Autodesk Fusion 360 part; units mm, degrees
(part 7 of 7)
  spline S53 degree 5 poles (-12.3121, 39.5225) (-12.3132, 39.5068) (-12.3154, 39.4756) (-12.3186, 39.4286) (-12.3227, 39.3661) (-12.3275, 39.288) (-12.332, 39.21) (-12.3361, 39.132) (-12.34, 39.054) (-12.3435, 38.9761) (-12.3467, 38.8983) (-12.3495, 38.8205) (-12.3521, 38.7428) (-12.3543, 38.6651) (-12.3562, 38.5875) (-12.3578, 38.51) (-12.359, 38.4325) (-12.3599, 38.3551) (-12.3605, 38.2777) (-12.3607, 38.2004) (-12.3606, 38.1232) (-12.3601, 38.0461) (-12.3593, 37.969) (-12.3581, 37.892) (-12.3566, 37.8151) (-12.3548, 37.7383) (-12.3525, 37.6615) (-12.35, 37.5848) (-12.347, 37.5082) (-12.3437, 37.4317) (-12.34, 37.3553) (-12.336, 37.2789) (-12.3315, 37.2027) (-12.3267, 37.1265) (-12.3215, 37.0505) (-12.3159, 36.9745) (-12.3099, 36.8987) (-12.3036, 36.8229) (-12.2968, 36.7473) (-12.2896, 36.6717) (-12.282, 36.5963) (-12.274, 36.521) (-12.2656, 36.4458) (-12.2567, 36.3708) (-12.2474, 36.2958) (-12.2377, 36.221) (-12.2275, 36.1463) (-12.2169, 36.0718) (-12.2059, 35.9974) (-12.1944, 35.9231) (-12.1823, 35.849) (-12.1698, 35.775) (-12.1568, 35.7013) (-12.1432, 35.6277) (-12.1291, 35.5542) (-12.1145, 35.481) (-12.0994, 35.4079) (-12.0838, 35.3349) (-12.0678, 35.2622) (-12.0511, 35.1896) (-12.0338, 35.1173) (-12.0157, 35.0453) (-11.9967, 34.9736) (-11.9769, 34.9022) (-11.9563, 34.8311) (-11.9352, 34.7603) (-11.9136, 34.6896) (-11.8917, 34.619) (-11.8692, 34.5488) (-11.8455, 34.4789) (-11.8201, 34.4098) (-11.7979, 34.3554) (-11.7798, 34.3151) (-11.7671, 34.2886) (-11.7607, 34.2754) knots -1 -1 -1 -1 -1 -1 -0.98571429 -0.97142857 -0.95714286 -0.94285714 -0.92857143 -0.91428571 -0.9 -0.88571429 -0.87142857 -0.85714286 -0.84285714 -0.82857143 -0.81428571 -0.8 -0.78571429 -0.77142857 -0.75714286 -0.74285714 -0.72857143 -0.71428571 -0.7 -0.68571429 -0.67142857 -0.65714286 -0.64285714 -0.62857143 -0.61428571 -0.6 -0.58571429 -0.57142857 -0.55714286 -0.54285714 -0.52857143 -0.51428571 -0.5 -0.48571429 -0.47142857 -0.45714286 -0.44285714 -0.42857143 -0.41428571 -0.4 -0.38571429 -0.37142857 -0.35714286 -0.34285714 -0.32857143 -0.31428571 -0.3 -0.28571429 -0.27142857 -0.25714286 -0.24285714 -0.22857143 -0.21428571 -0.2 -0.18571429 -0.17142857 -0.15714286 -0.14285714 -0.12857143 -0.11428571 -0.1 -0.08571429 -0.07142857 -0.05714286 -0.04285714 -0.02857143 -0.01428571 0 0 0 0 0 0
  line L53 (-11.7607, 34.2754) -> (-11.6323, 34.014)
  arc A108 (-11.7749, 33.5903) -> (-11.6323, 34.014) centre (-11.9173, 33.8741) ccw
  arc A109 (-11.7749, 33.5903) -> (-13.4852, 32.6761) centre (5.08, 0) ccw
  arc A110 (-13.9168, 32.7929) -> (-13.4852, 32.6761) centre (-13.6421, 32.9522) ccw
  line L54 (-13.9168, 32.7929) -> (-14.0628, 33.0449)
  spline S54 degree 5 poles (-14.0628, 33.0449) (-14.0701, 33.0576) (-14.0852, 33.0829) (-14.1086, 33.1203) (-14.1415, 33.169) (-14.1849, 33.2285) (-14.2298, 33.287) (-14.2757, 33.3448) (-14.3222, 33.4022) (-14.369, 33.4594) (-14.4162, 33.5163) (-14.4638, 33.5729) (-14.5121, 33.6291) (-14.5612, 33.6847) (-14.611, 33.7397) (-14.6615, 33.7943) (-14.7126, 33.8485) (-14.7642, 33.9022) (-14.8162, 33.9557) (-14.8686, 34.0089) (-14.9214, 34.0617) (-14.9746, 34.1142) (-15.0283, 34.1664) (-15.0824, 34.2183) (-15.1369, 34.2698) (-15.1919, 34.3209) (-15.2472, 34.3717) (-15.303, 34.4223) (-15.359, 34.4725) (-15.4155, 34.5225) (-15.4723, 34.5721) (-15.5294, 34.6215) (-15.5869, 34.6706) (-15.6447, 34.7193) (-15.7029, 34.7678) (-15.7614, 34.816) (-15.8202, 34.864) (-15.8794, 34.9116) (-15.9388, 34.959) (-15.9985, 35.0061) (-16.0586, 35.053) (-16.1189, 35.0995) (-16.1796, 35.1459) (-16.2405, 35.1919) (-16.3017, 35.2377) (-16.3632, 35.2832) (-16.425, 35.3285) (-16.4871, 35.3735) (-16.5494, 35.4182) (-16.612, 35.4627) (-16.6748, 35.507) (-16.738, 35.551) (-16.8013, 35.5947) (-16.865, 35.6382) (-16.9288, 35.6814) (-16.993, 35.7244) (-17.0574, 35.7672) (-17.122, 35.8097) (-17.1869, 35.852) (-17.252, 35.894) (-17.3173, 35.9358) (-17.3829, 35.9773) (-17.4487, 36.0186) (-17.5148, 36.0597) (-17.581, 36.1005) (-17.6475, 36.1411) (-17.7142, 36.1814) (-17.7812, 36.2215) (-17.8483, 36.2614) (-17.9157, 36.3011) (-17.9833, 36.3405) (-18.0376, 36.3718) (-18.0783, 36.3952) (-18.1056, 36.4108) (-18.1192, 36.4185) knots 0 0 0 0 0 0 0.01428571 0.02857143 0.04285714 0.05714286 0.07142857 0.08571429 0.1 0.11428571 0.12857143 0.14285714 0.15714286 0.17142857 0.18571429 0.2 0.21428571 0.22857143 0.24285714 0.25714286 0.27142857 0.28571429 0.3 0.31428571 0.32857143 0.34285714 0.35714286 0.37142857 0.38571429 0.4 0.41428571 0.42857143 0.44285714 0.45714286 0.47142857 0.48571429 0.5 0.51428571 0.52857143 0.54285714 0.55714286 0.57142857 0.58571429 0.6 0.61428571 0.62857143 0.64285714 0.65714286 0.67142857 0.68571429 0.7 0.71428571 0.72857143 0.74285714 0.75714286 0.77142857 0.78571429 0.8 0.81428571 0.82857143 0.84285714 0.85714286 0.87142857 0.88571429 0.9 0.91428571 0.92857143 0.94285714 0.95714286 0.97142857 0.98571429 1 1 1 1 1 1
  arc A111 (-18.1192, 36.4185) -> (-19.6884, 35.37) centre (5.08, 0) ccw
  spline S55 degree 5 poles (-19.6884, 35.37) (-19.6864, 35.3545) (-19.6825, 35.3234) (-19.6765, 35.2767) (-19.6683, 35.2146) (-19.6577, 35.1371) (-19.6469, 35.0597) (-19.6357, 34.9824) (-19.6243, 34.9052) (-19.6126, 34.8281) (-19.6005, 34.7511) (-19.5882, 34.6743) (-19.5755, 34.5975) (-19.5625, 34.5209) (-19.5492, 34.4444) (-19.5356, 34.3681) (-19.5217, 34.2918) (-19.5075, 34.2157) (-19.493, 34.1398) (-19.4781, 34.0639) (-19.4629, 33.9882) (-19.4474, 33.9126) (-19.4316, 33.8372) (-19.4154, 33.7619) (-19.3989, 33.6868) (-19.3821, 33.6118) (-19.365, 33.5369) (-19.3475, 33.4622) (-19.3296, 33.3877) (-19.3115, 33.3133) (-19.2929, 33.239) (-19.2741, 33.1649) (-19.2548, 33.091) (-19.2353, 33.0173) (-19.2153, 32.9437) (-19.195, 32.8703) (-19.1744, 32.7971) (-19.1533, 32.724) (-19.1319, 32.6511) (-19.1102, 32.5785) (-19.088, 32.506) (-19.0655, 32.4337) (-19.0425, 32.3616) (-19.0192, 32.2897) (-18.9954, 32.218) (-18.9713, 32.1465) (-18.9468, 32.0753) (-18.9218, 32.0042) (-18.8965, 31.9334) (-18.8707, 31.8628) (-18.8444, 31.7924) (-18.8177, 31.7224) (-18.7906, 31.6525) (-18.7629, 31.583) (-18.7347, 31.5137) (-18.7061, 31.4447) (-18.677, 31.376) (-18.6475, 31.3075) (-18.6176, 31.2392) (-18.5871, 31.1713) (-18.556, 31.1038) (-18.5242, 31.0367) (-18.4916, 30.9701) (-18.4582, 30.9039) (-18.4242, 30.8382) (-18.3896, 30.7729) (-18.3547, 30.7077) (-18.3194, 30.6428) (-18.2836, 30.5783) (-18.2468, 30.5144) (-18.2084, 30.4516) (-18.176, 30.4026) (-18.1504, 30.3666) (-18.1328, 30.343) (-18.1239, 30.3313) knots -1 -1 -1 -1 -1 -1 -0.98571429 -0.97142857 -0.95714286 -0.94285714 -0.92857143 -0.91428571 -0.9 -0.88571429 -0.87142857 -0.85714286 -0.84285714 -0.82857143 -0.81428571 -0.8 -0.78571429 -0.77142857 -0.75714286 -0.74285714 -0.72857143 -0.71428571 -0.7 -0.68571429 -0.67142857 -0.65714286 -0.64285714 -0.62857143 -0.61428571 -0.6 -0.58571429 -0.57142857 -0.55714286 -0.54285714 -0.52857143 -0.51428571 -0.5 -0.48571429 -0.47142857 -0.45714286 -0.44285714 -0.42857143 -0.41428571 -0.4 -0.38571429 -0.37142857 -0.35714286 -0.34285714 -0.32857143 -0.31428571 -0.3 -0.28571429 -0.27142857 -0.25714286 -0.24285714 -0.22857143 -0.21428571 -0.2 -0.18571429 -0.17142857 -0.15714286 -0.14285714 -0.12857143 -0.11428571 -0.1 -0.08571429 -0.07142857 -0.05714286 -0.04285714 -0.02857143 -0.01428571 0 0 0 0 0 0
  line L55 (-18.1239, 30.3313) -> (-17.947, 30.1)
  arc A112 (-18.0042, 29.6566) -> (-17.947, 30.1) centre (-18.1992, 29.9072) ccw
  arc A113 (-18.0042, 29.6566) -> (-19.5033, 28.4263) centre (5.08, 0) ccw
  arc A114 (-19.9493, 28.4568) -> (-19.5033, 28.4263) centre (-19.711, 28.6665) ccw
  line L56 (-19.9493, 28.4568) -> (-20.1417, 28.6753)
  spline S56 degree 5 poles (-20.1417, 28.6753) (-20.1514, 28.6864) (-20.1711, 28.7083) (-20.2014, 28.7404) (-20.2431, 28.7818) (-20.2972, 28.8317) (-20.3527, 28.8802) (-20.409, 28.9279) (-20.4658, 28.9752) (-20.5229, 29.0222) (-20.5803, 29.0688) (-20.638, 29.115) (-20.6964, 29.1607) (-20.7554, 29.2056) (-20.815, 29.2499) (-20.8751, 29.2936) (-20.9358, 29.3367) (-20.9969, 29.3794) (-21.0584, 29.4217) (-21.1201, 29.4636) (-21.1822, 29.5051) (-21.2446, 29.5463) (-21.3074, 29.587) (-21.3706, 29.6273) (-21.4341, 29.6671) (-21.498, 29.7066) (-21.5622, 29.7457) (-21.6268, 29.7843) (-21.6916, 29.8227) (-21.7567, 29.8606) (-21.8221, 29.8983) (-21.8877, 29.9355) (-21.9537, 29.9725) (-22.0199, 30.009) (-22.0864, 30.0452) (-22.1532, 30.0811) (-22.2203, 30.1166) (-22.2875, 30.1518) (-22.3551, 30.1867) (-22.4229, 30.2213) (-22.4909, 30.2555) (-22.5592, 30.2894) (-22.6277, 30.323) (-22.6964, 30.3563) (-22.7654, 30.3892) (-22.8346, 30.4219) (-22.904, 30.4542) (-22.9737, 30.4863) (-23.0435, 30.518) (-23.1136, 30.5494) (-23.1839, 30.5806) (-23.2544, 30.6114) (-23.3251, 30.6419) (-23.396, 30.6722) (-23.4671, 30.7021) (-23.5383, 30.7318) (-23.6098, 30.7612) (-23.6815, 30.7902) (-23.7534, 30.819) (-23.8254, 30.8475) (-23.8977, 30.8758) (-23.9701, 30.9037) (-24.0427, 30.9314) (-24.1155, 30.9588) (-24.1885, 30.9859) (-24.2616, 31.0127) (-24.3349, 31.0393) (-24.4084, 31.0656) (-24.482, 31.0916) (-24.5558, 31.1173) (-24.6298, 31.1428) (-24.6891, 31.1629) (-24.7337, 31.1779) (-24.7635, 31.1879) (-24.7783, 31.1928) knots 0 0 0 0 0 0 0.01428571 0.02857143 0.04285714 0.05714286 0.07142857 0.08571429 0.1 0.11428571 0.12857143 0.14285714 0.15714286 0.17142857 0.18571429 0.2 0.21428571 0.22857143 0.24285714 0.25714286 0.27142857 0.28571429 0.3 0.31428571 0.32857143 0.34285714 0.35714286 0.37142857 0.38571429 0.4 0.41428571 0.42857143 0.44285714 0.45714286 0.47142857 0.48571429 0.5 0.51428571 0.52857143 0.54285714 0.55714286 0.57142857 0.58571429 0.6 0.61428571 0.62857143 0.64285714 0.65714286 0.67142857 0.68571429 0.7 0.71428571 0.72857143 0.74285714 0.75714286 0.77142857 0.78571429 0.8 0.81428571 0.82857143 0.84285714 0.85714286 0.87142857 0.88571429 0.9 0.91428571 0.92857143 0.94285714 0.95714286 0.97142857 0.98571429 1 1 1 1 1 1
  arc A115 (-24.7783, 31.1928) -> (-26.1128, 29.8583) centre (5.08, 0) ccw
  spline S57 degree 5 poles (-26.1128, 29.8583) (-26.1079, 29.8435) (-26.0979, 29.8137) (-26.0829, 29.7691) (-26.0628, 29.7098) (-26.0373, 29.6358) (-26.0116, 29.562) (-25.9856, 29.4884) (-25.9593, 29.4149) (-25.9327, 29.3416) (-25.9059, 29.2685) (-25.8788, 29.1955) (-25.8514, 29.1227) (-25.8237, 29.0501) (-25.7958, 28.9777) (-25.7675, 28.9054) (-25.739, 28.8334) (-25.7102, 28.7615) (-25.6812, 28.6898) (-25.6518, 28.6183) (-25.6221, 28.5471) (-25.5922, 28.476) (-25.5619, 28.4051) (-25.5314, 28.3344) (-25.5006, 28.2639) (-25.4694, 28.1936) (-25.438, 28.1235) (-25.4063, 28.0537) (-25.3742, 27.984) (-25.3419, 27.9146) (-25.3092, 27.8454) (-25.2763, 27.7764) (-25.243, 27.7077) (-25.2094, 27.6392) (-25.1755, 27.5709) (-25.1413, 27.5029) (-25.1067, 27.4351) (-25.0718, 27.3675) (-25.0366, 27.3003) (-25.0011, 27.2332) (-24.9652, 27.1664) (-24.929, 27.0999) (-24.8925, 27.0337) (-24.8555, 26.9677) (-24.8183, 26.9021) (-24.7806, 26.8367) (-24.7427, 26.7716) (-24.7043, 26.7068) (-24.6657, 26.6422) (-24.6266, 26.578) (-24.5871, 26.5141) (-24.5473, 26.4506) (-24.507, 26.3874) (-24.4663, 26.3246) (-24.4251, 26.2622) (-24.3836, 26.2001) (-24.3417, 26.1384) (-24.2994, 26.0769) (-24.2567, 26.0158) (-24.2136, 25.9551) (-24.1699, 25.895) (-24.1256, 25.8354) (-24.0807, 25.7764) (-24.035, 25.718) (-23.9888, 25.6603) (-23.9422, 25.6029) (-23.8952, 25.5458) (-23.8479, 25.489) (-23.8002, 25.4327) (-23.7517, 25.3772) (-23.7018, 25.3231) (-23.6604, 25.2814) (-23.6283, 25.2511) (-23.6064, 25.2314) (-23.5953, 25.2217) knots -1 -1 -1 -1 -1 -1 -0.98571429 -0.97142857 -0.95714286 -0.94285714 -0.92857143 -0.91428571 -0.9 -0.88571429 -0.87142857 -0.85714286 -0.84285714 -0.82857143 -0.81428571 -0.8 -0.78571429 -0.77142857 -0.75714286 -0.74285714 -0.72857143 -0.71428571 -0.7 -0.68571429 -0.67142857 -0.65714286 -0.64285714 -0.62857143 -0.61428571 -0.6 -0.58571429 -0.57142857 -0.55714286 -0.54285714 -0.52857143 -0.51428571 -0.5 -0.48571429 -0.47142857 -0.45714286 -0.44285714 -0.42857143 -0.41428571 -0.4 -0.38571429 -0.37142857 -0.35714286 -0.34285714 -0.32857143 -0.31428571 -0.3 -0.28571429 -0.27142857 -0.25714286 -0.24285714 -0.22857143 -0.21428571 -0.2 -0.18571429 -0.17142857 -0.15714286 -0.14285714 -0.12857143 -0.11428571 -0.1 -0.08571429 -0.07142857 -0.05714286 -0.04285714 -0.02857143 -0.01428571 0 0 0 0 0 0
  line L57 (-23.5953, 25.2217) -> (-23.3768, 25.0293)
  arc A116 (-23.3463, 24.5833) -> (-23.3768, 25.0293) centre (-23.5865, 24.791) ccw
  arc A117 (-23.3463, 24.5833) -> (-24.5766, 23.0842) centre (5.08, 0) ccw
  arc A118 (-25.02, 23.027) -> (-24.5766, 23.0842) centre (-24.8272, 23.2792) ccw
  line L58 (-25.02, 23.027) -> (-25.2513, 23.2039)
  spline S58 degree 5 poles (-25.2513, 23.2039) (-25.263, 23.2128) (-25.2866, 23.2304) (-25.3226, 23.256) (-25.3716, 23.2884) (-25.4344, 23.3268) (-25.4983, 23.3636) (-25.5628, 23.3994) (-25.6277, 23.4347) (-25.6929, 23.4696) (-25.7582, 23.5042) (-25.8239, 23.5382) (-25.8901, 23.5716) (-25.9567, 23.6042) (-26.0238, 23.636) (-26.0913, 23.6671) (-26.1592, 23.6976) (-26.2275, 23.7275) (-26.296, 23.757) (-26.3647, 23.7861) (-26.4337, 23.8147) (-26.503, 23.8429) (-26.5725, 23.8706) (-26.6424, 23.8977) (-26.7124, 23.9244) (-26.7828, 23.9507) (-26.8534, 23.9765) (-26.9242, 24.0018) (-26.9953, 24.0268) (-27.0665, 24.0513) (-27.138, 24.0754) (-27.2097, 24.0992) (-27.2816, 24.1225) (-27.3537, 24.1455) (-27.426, 24.168) (-27.4985, 24.1902) (-27.5711, 24.2119) (-27.644, 24.2333) (-27.7171, 24.2544) (-27.7903, 24.275) (-27.8637, 24.2953) (-27.9373, 24.3153) (-28.011, 24.3348) (-28.0849, 24.3541) (-28.159, 24.3729) (-28.2333, 24.3915) (-28.3077, 24.4096) (-28.3822, 24.4275) (-28.4569, 24.445) (-28.5318, 24.4621) (-28.6068, 24.4789) (-28.6819, 24.4954) (-28.7572, 24.5116) (-28.8326, 24.5274) (-28.9082, 24.5429) (-28.9839, 24.5581) (-29.0598, 24.573) (-29.1357, 24.5875) (-29.2118, 24.6017) (-29.2881, 24.6156) (-29.3644, 24.6292) (-29.4409, 24.6425) (-29.5175, 24.6555) (-29.5943, 24.6682) (-29.6711, 24.6805) (-29.7481, 24.6926) (-29.8252, 24.7043) (-29.9024, 24.7157) (-29.9797, 24.7269) (-30.0571, 24.7377) (-30.1346, 24.7483) (-30.1967, 24.7565) (-30.2434, 24.7625) (-30.2745, 24.7664) (-30.29, 24.7684) knots 0 0 0 0 0 0 0.01428571 0.02857143 0.04285714 0.05714286 0.07142857 0.08571429 0.1 0.11428571 0.12857143 0.14285714 0.15714286 0.17142857 0.18571429 0.2 0.21428571 0.22857143 0.24285714 0.25714286 0.27142857 0.28571429 0.3 0.31428571 0.32857143 0.34285714 0.35714286 0.37142857 0.38571429 0.4 0.41428571 0.42857143 0.44285714 0.45714286 0.47142857 0.48571429 0.5 0.51428571 0.52857143 0.54285714 0.55714286 0.57142857 0.58571429 0.6 0.61428571 0.62857143 0.64285714 0.65714286 0.67142857 0.68571429 0.7 0.71428571 0.72857143 0.74285714 0.75714286 0.77142857 0.78571429 0.8 0.81428571 0.82857143 0.84285714 0.85714286 0.87142857 0.88571429 0.9 0.91428571 0.92857143 0.94285714 0.95714286 0.97142857 0.98571429 1 1 1 1 1 1
  arc A119 (-30.29, 24.7684) -> (-31.3385, 23.1992) centre (5.08, 0) ccw
  spline S59 degree 5 poles (-31.3385, 23.1992) (-31.3308, 23.1856) (-31.3152, 23.1583) (-31.2918, 23.1176) (-31.2605, 23.0633) (-31.2211, 22.9957) (-31.1814, 22.9283) (-31.1415, 22.8612) (-31.1014, 22.7942) (-31.0611, 22.7275) (-31.0205, 22.661) (-30.9797, 22.5948) (-30.9386, 22.5287) (-30.8973, 22.4629) (-30.8558, 22.3973) (-30.814, 22.332) (-30.772, 22.2669) (-30.7297, 22.202) (-30.6872, 22.1374) (-30.6444, 22.073) (-30.6014, 22.0088) (-30.5582, 21.945) (-30.5147, 21.8813) (-30.471, 21.818) (-30.427, 21.7548) (-30.3827, 21.692) (-30.3382, 21.6294) (-30.2935, 21.5671) (-30.2485, 21.505) (-30.2032, 21.4432) (-30.1577, 21.3817) (-30.1119, 21.3205) (-30.0659, 21.2596) (-30.0195, 21.1989) (-29.973, 21.1386) (-29.9261, 21.0785) (-29.879, 21.0188) (-29.8316, 20.9594) (-29.784, 20.9002) (-29.736, 20.8414) (-29.6878, 20.7829) (-29.6393, 20.7247) (-29.5906, 20.6669) (-29.5415, 20.6094) (-29.4921, 20.5523) (-29.4425, 20.4955) (-29.3925, 20.439) (-29.3423, 20.383) (-29.2917, 20.3272) (-29.2409, 20.2719) (-29.1898, 20.2169) (-29.1383, 20.1624) (-29.0864, 20.1083) (-29.0342, 20.0546) (-28.9817, 20.0014) (-28.9289, 19.9486) (-28.8757, 19.8962) (-28.8222, 19.8442) (-28.7685, 19.7926) (-28.7143, 19.7415) (-28.6597, 19.691) (-28.6047, 19.6412) (-28.5491, 19.5921) (-28.4929, 19.5438) (-28.4363, 19.4962) (-28.3794, 19.449) (-28.3222, 19.4022) (-28.2648, 19.3557) (-28.207, 19.3098) (-28.1485, 19.2649) (-28.089, 19.2215) (-28.0403, 19.1886) (-28.0029, 19.1652) (-27.9776, 19.1501) (-27.9649, 19.1428) knots -1 -1 -1 -1 -1 -1 -0.98571429 -0.97142857 -0.95714286 -0.94285714 -0.92857143 -0.91428571 -0.9 -0.88571429 -0.87142857 -0.85714286 -0.84285714 -0.82857143 -0.81428571 -0.8 -0.78571429 -0.77142857 -0.75714286 -0.74285714 -0.72857143 -0.71428571 -0.7 -0.68571429 -0.67142857 -0.65714286 -0.64285714 -0.62857143 -0.61428571 -0.6 -0.58571429 -0.57142857 -0.55714286 -0.54285714 -0.52857143 -0.51428571 -0.5 -0.48571429 -0.47142857 -0.45714286 -0.44285714 -0.42857143 -0.41428571 -0.4 -0.38571429 -0.37142857 -0.35714286 -0.34285714 -0.32857143 -0.31428571 -0.3 -0.28571429 -0.27142857 -0.25714286 -0.24285714 -0.22857143 -0.21428571 -0.2 -0.18571429 -0.17142857 -0.15714286 -0.14285714 -0.12857143 -0.11428571 -0.1 -0.08571429 -0.07142857 -0.05714286 -0.04285714 -0.02857143 -0.01428571 0 0 0 0 0 0
  line L59 (-27.9649, 19.1428) -> (-27.7129, 18.9968)
  arc A120 (-27.5961, 18.5652) -> (-27.7129, 18.9968) centre (-27.8722, 18.7221) ccw
  arc A121 (-27.5961, 18.5652) -> (-28.5103, 16.8549) centre (5.08, 0) ccw
  arc A122 (-28.934, 16.7123) -> (-28.5103, 16.8549) centre (-28.7941, 16.9973) ccw
  line L60 (-28.934, 16.7123) -> (-29.1954, 16.8407)
  spline S60 degree 5 poles (-29.1954, 16.8407) (-29.2086, 16.8471) (-29.2351, 16.8598) (-29.2754, 16.8779) (-29.3298, 16.9001) (-29.3989, 16.9255) (-29.4688, 16.9492) (-29.539, 16.9717) (-29.6096, 16.9936) (-29.6803, 17.0152) (-29.7511, 17.0363) (-29.8222, 17.0569) (-29.8936, 17.0767) (-29.9653, 17.0957) (-30.0373, 17.1138) (-30.1096, 17.1311) (-30.1822, 17.1478) (-30.2549, 17.1638) (-30.3279, 17.1794) (-30.401, 17.1945) (-30.4742, 17.2091) (-30.5477, 17.2232) (-30.6213, 17.2368) (-30.695, 17.2498) (-30.769, 17.2623) (-30.8431, 17.2744) (-30.9174, 17.2859) (-30.9918, 17.2969) (-31.0663, 17.3075) (-31.141, 17.3177) (-31.2158, 17.3274) (-31.2908, 17.3367) (-31.3658, 17.3456) (-31.441, 17.354) (-31.5163, 17.362) (-31.5917, 17.3696) (-31.6673, 17.3768) (-31.7429, 17.3836) (-31.8187, 17.3899) (-31.8945, 17.3959) (-31.9705, 17.4015) (-32.0465, 17.4067) (-32.1227, 17.4115) (-32.1989, 17.416) (-32.2753, 17.42) (-32.3517, 17.4237) (-32.4282, 17.427) (-32.5048, 17.43) (-32.5815, 17.4325) (-32.6583, 17.4348) (-32.7351, 17.4366) (-32.812, 17.4381) (-32.889, 17.4393) (-32.9661, 17.4401) (-33.0432, 17.4406) (-33.1204, 17.4407) (-33.1977, 17.4405) (-33.2751, 17.4399) (-33.3525, 17.439) (-33.43, 17.4378) (-33.5075, 17.4362) (-33.5851, 17.4343) (-33.6628, 17.4321) (-33.7405, 17.4295) (-33.8183, 17.4267) (-33.8961, 17.4235) (-33.974, 17.42) (-34.052, 17.4161) (-34.13, 17.412) (-34.208, 17.4075) (-34.2861, 17.4027) (-34.3486, 17.3986) (-34.3956, 17.3954) (-34.4268, 17.3932) (-34.4425, 17.3921) knots 0 0 0 0 0 0 0.01428571 0.02857143 0.04285714 0.05714286 0.07142857 0.08571429 0.1 0.11428571 0.12857143 0.14285714 0.15714286 0.17142857 0.18571429 0.2 0.21428571 0.22857143 0.24285714 0.25714286 0.27142857 0.28571429 0.3 0.31428571 0.32857143 0.34285714 0.35714286 0.37142857 0.38571429 0.4 0.41428571 0.42857143 0.44285714 0.45714286 0.47142857 0.48571429 0.5 0.51428571 0.52857143 0.54285714 0.55714286 0.57142857 0.58571429 0.6 0.61428571 0.62857143 0.64285714 0.65714286 0.67142857 0.68571429 0.7 0.71428571 0.72857143 0.74285714 0.75714286 0.77142857 0.78571429 0.8 0.81428571 0.82857143 0.84285714 0.85714286 0.87142857 0.88571429 0.9 0.91428571 0.92857143 0.94285714 0.95714286 0.97142857 0.98571429 1 1 1 1 1 1
  arc A123 (-34.4425, 17.3921) -> (-35.1647, 15.6485) centre (5.08, 0) ccw
  spline S61 degree 5 poles (-35.1647, 15.6485) (-35.1544, 15.6367) (-35.1339, 15.613) (-35.103, 15.5776) (-35.0616, 15.5305) (-35.0098, 15.4719) (-34.9578, 15.4135) (-34.9055, 15.3554) (-34.8531, 15.2976) (-34.8006, 15.24) (-34.7478, 15.1827) (-34.6948, 15.1257) (-34.6417, 15.0689) (-34.5883, 15.0125) (-34.5348, 14.9562) (-34.481, 14.9003) (-34.4271, 14.8446) (-34.373, 14.7893) (-34.3187, 14.7342) (-34.2642, 14.6794) (-34.2095, 14.6248) (-34.1547, 14.5706) (-34.0996, 14.5167) (-34.0443, 14.4631) (-33.9889, 14.4098) (-33.9332, 14.3567) (-33.8774, 14.304) (-33.8213, 14.2516) (-33.7651, 14.1996) (-33.7086, 14.1478) (-33.652, 14.0964) (-33.5951, 14.0452) (-33.5381, 13.9945) (-33.4808, 13.944) (-33.4234, 13.8939) (-33.3657, 13.8442) (-33.3078, 13.7948) (-33.2498, 13.7457) (-33.1915, 13.697) (-33.133, 13.6487) (-33.0743, 13.6007) (-33.0154, 13.5531) (-32.9563, 13.5059) (-32.8969, 13.4591) (-32.8374, 13.4127) (-32.7776, 13.3667) (-32.7176, 13.3211) (-32.6574, 13.2758) (-32.5969, 13.231) (-32.5363, 13.1867) (-32.4754, 13.1427) (-32.4142, 13.0993) (-32.3529, 13.0564) (-32.2912, 13.0139) (-32.2293, 12.972) (-32.1672, 12.9305) (-32.1048, 12.8895) (-32.0422, 12.8489) (-31.9794, 12.8088) (-31.9164, 12.7693) (-31.853, 12.7304) (-31.7892, 12.6922) (-31.7251, 12.655) (-31.6606, 12.6185) (-31.5958, 12.5828) (-31.5308, 12.5477) (-31.4656, 12.5129) (-31.4002, 12.4786) (-31.3345, 12.4448) (-31.2684, 12.4121) (-31.2016, 12.3812) (-31.1474, 12.3585) (-31.1062, 12.3428) (-31.0784, 12.333) (-31.0645, 12.3282) knots -1 -1 -1 -1 -1 -1 -0.98571429 -0.97142857 -0.95714286 -0.94285714 -0.92857143 -0.91428571 -0.9 -0.88571429 -0.87142857 -0.85714286 -0.84285714 -0.82857143 -0.81428571 -0.8 -0.78571429 -0.77142857 -0.75714286 -0.74285714 -0.72857143 -0.71428571 -0.7 -0.68571429 -0.67142857 -0.65714286 -0.64285714 -0.62857143 -0.61428571 -0.6 -0.58571429 -0.57142857 -0.55714286 -0.54285714 -0.52857143 -0.51428571 -0.5 -0.48571429 -0.47142857 -0.45714286 -0.44285714 -0.42857143 -0.41428571 -0.4 -0.38571429 -0.37142857 -0.35714286 -0.34285714 -0.32857143 -0.31428571 -0.3 -0.28571429 -0.27142857 -0.25714286 -0.24285714 -0.22857143 -0.21428571 -0.2 -0.18571429 -0.17142857 -0.15714286 -0.14285714 -0.12857143 -0.11428571 -0.1 -0.08571429 -0.07142857 -0.05714286 -0.04285714 -0.02857143 -0.01428571 0 0 0 0 0 0
  line L61 (-31.0645, 12.3282) -> (-30.7889, 12.2341)
  arc A124 (-30.5901, 11.8337) -> (-30.7889, 12.2341) centre (-30.8915, 11.9337) ccw
  arc A125 (-30.5901, 11.8337) -> (-31.1531, 9.9779) centre (5.08, 0) ccw
  arc A126 (-31.5408, 9.7554) -> (-31.1531, 9.9779) centre (-31.4592, 10.0622) ccw
  line L62 (-31.5408, 9.7554) -> (-31.8222, 9.8303)
  spline S62 degree 5 poles (-31.8222, 9.8303) (-31.8364, 9.8341) (-31.865, 9.8413) (-31.908, 9.8512) (-31.9657, 9.8624) (-32.0384, 9.8738) (-32.1115, 9.8834) (-32.1849, 9.8917) (-32.2583, 9.8995) (-32.3319, 9.9069) (-32.4055, 9.9138) (-32.4792, 9.9201) (-32.5531, 9.9256) (-32.6271, 9.9302) (-32.7013, 9.934) (-32.7756, 9.9368) (-32.85, 9.939) (-32.9245, 9.9405) (-32.9991, 9.9416) (-33.0737, 9.9421) (-33.1484, 9.9421) (-33.2232, 9.9416) (-33.298, 9.9406) (-33.3729, 9.939) (-33.4479, 9.9369) (-33.5229, 9.9342) (-33.598, 9.931) (-33.6731, 9.9273) (-33.7483, 9.9232) (-33.8236, 9.9186) (-33.8988, 9.9135) (-33.9741, 9.908) (-34.0495, 9.9021) (-34.1249, 9.8957) (-34.2003, 9.8888) (-34.2758, 9.8816) (-34.3512, 9.8739) (-34.4268, 9.8657) (-34.5023, 9.8572) (-34.5779, 9.8483) (-34.6534, 9.8389) (-34.729, 9.8292) (-34.8047, 9.8191) (-34.8803, 9.8086) (-34.956, 9.7976) (-35.0316, 9.7863) (-35.1073, 9.7747) (-35.183, 9.7626) (-35.2588, 9.7502) (-35.3345, 9.7374) (-35.4102, 9.7242) (-35.4859, 9.7107) (-35.5617, 9.6968) (-35.6374, 9.6826) (-35.7132, 9.668) (-35.7889, 9.653) (-35.8647, 9.6377) (-35.9405, 9.6221) (-36.0162, 9.6061) (-36.092, 9.5898) (-36.1677, 9.5731) (-36.2435, 9.5561) (-36.3192, 9.5388) (-36.3949, 9.5211) (-36.4707, 9.5031) (-36.5464, 9.4848) (-36.6221, 9.4662) (-36.6978, 9.4472) (-36.7735, 9.4279) (-36.8492, 9.4083) (-36.9248, 9.3884) (-36.9853, 9.3722) (-37.0307, 9.3599) (-37.061, 9.3516) (-37.0761, 9.3475) knots 0 0 0 0 0 0 0.01428571 0.02857143 0.04285714 0.05714286 0.07142857 0.08571429 0.1 0.11428571 0.12857143 0.14285714 0.15714286 0.17142857 0.18571429 0.2 0.21428571 0.22857143 0.24285714 0.25714286 0.27142857 0.28571429 0.3 0.31428571 0.32857143 0.34285714 0.35714286 0.37142857 0.38571429 0.4 0.41428571 0.42857143 0.44285714 0.45714286 0.47142857 0.48571429 0.5 0.51428571 0.52857143 0.54285714 0.55714286 0.57142857 0.58571429 0.6 0.61428571 0.62857143 0.64285714 0.65714286 0.67142857 0.68571429 0.7 0.71428571 0.72857143 0.74285714 0.75714286 0.77142857 0.78571429 0.8 0.81428571 0.82857143 0.84285714 0.85714286 0.87142857 0.88571429 0.9 0.91428571 0.92857143 0.94285714 0.95714286 0.97142857 0.98571429 1 1 1 1 1 1
  arc A127 (-37.0761, 9.3475) -> (-37.4443, 7.4965) centre (5.08, 0) ccw
  spline S63 degree 5 poles (-37.4443, 7.4965) (-37.4319, 7.4869) (-37.4071, 7.4677) (-37.3699, 7.4389) (-37.3202, 7.4008) (-37.2579, 7.3535) (-37.1955, 7.3064) (-37.1329, 7.2596) (-37.0703, 7.2131) (-37.0074, 7.1669) (-36.9445, 7.121) (-36.8814, 7.0754) (-36.8182, 7.0301) (-36.7549, 6.9851) (-36.6914, 6.9404) (-36.6278, 6.896) (-36.5641, 6.8519) (-36.5002, 6.8082) (-36.4362, 6.7647) (-36.372, 6.7216) (-36.3078, 6.6788) (-36.2434, 6.6364) (-36.1788, 6.5942) (-36.1142, 6.5524) (-36.0494, 6.5109) (-35.9844, 6.4698) (-35.9194, 6.429) (-35.8542, 6.3885) (-35.7889, 6.3484) (-35.7234, 6.3087) (-35.6578, 6.2693) (-35.5921, 6.2302) (-35.5262, 6.1916) (-35.4602, 6.1533) (-35.3941, 6.1153) (-35.3279, 6.0778) (-35.2615, 6.0406) (-35.1949, 6.0038) (-35.1283, 5.9674) (-35.0615, 5.9314) (-34.9946, 5.8958) (-34.9275, 5.8606) (-34.8603, 5.8259) (-34.793, 5.7916) (-34.7255, 5.7577) (-34.6579, 5.7242) (-34.5901, 5.6912) (-34.5223, 5.6586) (-34.4542, 5.6264) (-34.3861, 5.5947) (-34.3178, 5.5635) (-34.2493, 5.5328) (-34.1808, 5.5027) (-34.112, 5.4731) (-34.0431, 5.444) (-33.9741, 5.4155) (-33.9049, 5.3874) (-33.8356, 5.3598) (-33.7662, 5.3328) (-33.6966, 5.3063) (-33.6269, 5.2805) (-33.5569, 5.2555) (-33.4868, 5.2315) (-33.4164, 5.2083) (-33.3459, 5.186) (-33.2753, 5.1642) (-33.2045, 5.1428) (-33.1336, 5.1219) (-33.0627, 5.1016) (-32.9915, 5.0824) (-32.9199, 5.0651) (-32.8623, 5.0534) (-32.8188, 5.0461) (-32.7897, 5.0418) (-32.7751, 5.0399) knots -1 -1 -1 -1 -1 -1 -0.98571429 -0.97142857 -0.95714286 -0.94285714 -0.92857143 -0.91428571 -0.9 -0.88571429 -0.87142857 -0.85714286 -0.84285714 -0.82857143 -0.81428571 -0.8 -0.78571429 -0.77142857 -0.75714286 -0.74285714 -0.72857143 -0.71428571 -0.7 -0.68571429 -0.67142857 -0.65714286 -0.64285714 -0.62857143 -0.61428571 -0.6 -0.58571429 -0.57142857 -0.55714286 -0.54285714 -0.52857143 -0.51428571 -0.5 -0.48571429 -0.47142857 -0.45714286 -0.44285714 -0.42857143 -0.41428571 -0.4 -0.38571429 -0.37142857 -0.35714286 -0.34285714 -0.32857143 -0.31428571 -0.3 -0.28571429 -0.27142857 -0.25714286 -0.24285714 -0.22857143 -0.21428571 -0.2 -0.18571429 -0.17142857 -0.15714286 -0.14285714 -0.12857143 -0.11428571 -0.1 -0.08571429 -0.07142857 -0.05714286 -0.04285714 -0.02857143 -0.01428571 0 0 0 0 0 0
  line L63 (-32.7751, 5.0399) -> (-32.4865, 5.0014)
  arc A128 (-32.2134, 4.6474) -> (-32.4865, 5.0014) centre (-32.5284, 4.6867) ccw
component "Spur Gear (32 teeth)" placed x (1, 0, 0) y (0, 1, 0) z (0, 0, 1) at (0, 0, 0)
equation "d13 = -2.54 mm + 10 mm"
